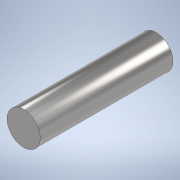
# Autodesk Inventor part: wheel_axle
Saved by Autodesk Inventor 2022 (Build 260153000, 153)
## iProperties
Created: 2021-11-07
Part Number: wheel_axle
Material: Steel, Alloy
Document SubType Name: Modeling
Designer: kibandi
Density: 7.73 g/cm^3
Appearance: Semi-Polished
Mass: 169.992 g
Surface Area: 50.2655 cm^2
Volume: 21.9911 cm^3
Author: kibandi
Autodesk Inventor part; units mm, degrees
ref_plane "YZ Plane" through (0, 0, 0) normal (1, 0, 0) x (0, 1, 0)
ref_plane "XZ Plane" through (0, 0, 0) normal (0, 1, 0) x (-1, 0, 0)
ref_plane "XY Plane" through (0, 0, 0) normal (0, 0, 1) x (1, 0, 0)
sketch "Sketch1" plane through (0, 0, 0) normal (0, 0, 1) x (1, 0, 0)
  circle A0 centre (0, 0) radius 10
  dimension "d0" = 20
  constraints: 1 centre point, 1 coincident
  measures "d0" diameter of A0
extrude "Extrusion1" add sketch "Sketch1" along normal blind 80
body "Solid1"
